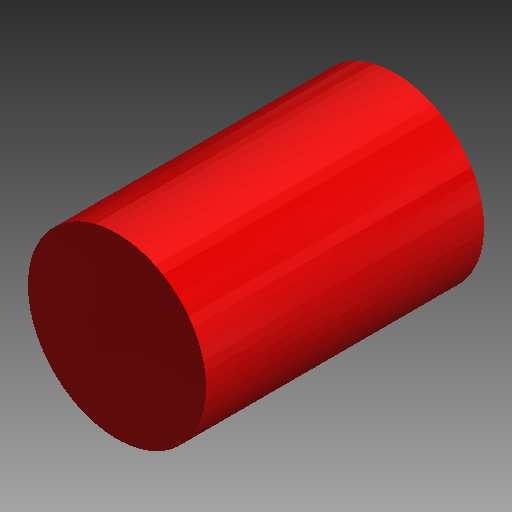
# Autodesk Inventor part: 470uF
Saved by Autodesk Inventor 2018.2 (Build 222227000, 227)
## iProperties
Part Number: 470uF
Material: Generic
Document SubType Name: Modeling
Designer: autocad
Appearance: C12,5-5, 470uF
Author: autocad
Autodesk Inventor part; units mm, degrees
ref_plane "YZ Plane" through (0, 0, 0) normal (1, 0, 0) x (0, 1, 0)
ref_plane "XZ Plane" through (0, 0, 0) normal (0, 1, 0) x (-1, 0, 0)
ref_plane "XY Plane" through (0, 0, 0) normal (0, 0, 1) x (1, 0, 0)
sketch "C12,5-5, 470uF_126" plane through (0, 0, 0) normal (0, 0, 1) x (1, 0, 0)
  line L0 (0.9403, 6.3386) -> (1.557, 6.216)
  line L1 (1.557, 6.216) -> (2.1588, 6.0334)
  line L2 (2.1588, 6.0334) -> (2.7398, 5.7928)
  line L3 (2.7398, 5.7928) -> (3.2944, 5.4963)
  line L4 (3.2944, 5.4963) -> (3.8172, 5.147)
  line L5 (3.8172, 5.147) -> (4.3033, 4.748)
  line L6 (4.3033, 4.748) -> (4.748, 4.3034)
  line L7 (4.748, 4.3034) -> (5.147, 3.8172)
  line L8 (5.147, 3.8172) -> (5.4963, 3.2944)
  line L9 (5.4963, 3.2944) -> (5.7928, 2.7398)
  line L10 (5.7928, 2.7398) -> (6.0334, 2.1588)
  line L11 (6.0334, 2.1588) -> (6.216, 1.557)
  line L12 (6.216, 1.557) -> (6.3386, 0.9403)
  line L13 (6.3386, 0.9403) -> (6.4003, 0.3144)
  line L14 (6.4003, 0.3144) -> (6.4003, 0)
  line L15 (6.4003, 0) -> (6.4003, -0.3144)
  line L16 (6.4003, -0.3144) -> (6.3386, -0.9403)
  line L17 (6.3386, -0.9403) -> (6.216, -1.557)
  line L18 (6.216, -1.557) -> (6.0334, -2.1588)
  line L19 (6.0334, -2.1588) -> (5.7928, -2.7398)
  line L20 (5.7928, -2.7398) -> (5.4963, -3.2944)
  line L21 (5.4963, -3.2944) -> (5.147, -3.8172)
  line L22 (5.147, -3.8172) -> (4.748, -4.3033)
  line L23 (4.748, -4.3033) -> (4.3033, -4.748)
  line L24 (4.3033, -4.748) -> (3.8172, -5.147)
  line L25 (3.8172, -5.147) -> (3.2944, -5.4963)
  line L26 (3.2944, -5.4963) -> (2.7398, -5.7928)
  line L27 (2.7398, -5.7928) -> (2.1588, -6.0334)
  line L28 (2.1588, -6.0334) -> (1.557, -6.216)
  line L29 (1.557, -6.216) -> (0.9403, -6.3386)
  line L30 (0.9403, -6.3386) -> (0.3144, -6.4003)
  line L31 (0.3144, -6.4003) -> (-0.3144, -6.4003)
  line L32 (-0.3144, -6.4003) -> (-0.9403, -6.3386)
  line L33 (-0.9403, -6.3386) -> (-1.557, -6.216)
  line L34 (-1.557, -6.216) -> (-2.1588, -6.0334)
  line L35 (-2.1588, -6.0334) -> (-2.7398, -5.7928)
  line L36 (-2.7398, -5.7928) -> (-3.2944, -5.4963)
  line L37 (-3.2944, -5.4963) -> (-3.8172, -5.147)
  line L38 (-3.8172, -5.147) -> (-4.3034, -4.748)
  line L39 (-4.3034, -4.748) -> (-4.748, -4.3033)
  line L40 (-4.748, -4.3033) -> (-5.147, -3.8172)
  line L41 (-5.147, -3.8172) -> (-5.4963, -3.2944)
  line L42 (-5.4963, -3.2944) -> (-5.7928, -2.7398)
  line L43 (-5.7928, -2.7398) -> (-6.0334, -2.1588)
  line L44 (-6.0334, -2.1588) -> (-6.216, -1.557)
  line L45 (-6.216, -1.557) -> (-6.3386, -0.9403)
  line L46 (-6.3386, -0.9403) -> (-6.4003, -0.3144)
  line L47 (-6.4003, -0.3144) -> (-6.4003, 0)
  line L48 (-6.4003, 0) -> (-6.4003, 0.3144)
  line L49 (-6.4003, 0.3144) -> (-6.3386, 0.9403)
  line L50 (-6.3386, 0.9403) -> (-6.216, 1.557)
  line L51 (-6.216, 1.557) -> (-6.0334, 2.1588)
  line L52 (-6.0334, 2.1588) -> (-5.7928, 2.7398)
  line L53 (-5.7928, 2.7398) -> (-5.4963, 3.2944)
  line L54 (-5.4963, 3.2944) -> (-5.147, 3.8172)
  line L55 (-5.147, 3.8172) -> (-4.748, 4.3034)
  line L56 (-4.748, 4.3034) -> (-4.3034, 4.748)
  line L57 (-4.3034, 4.748) -> (-3.8172, 5.147)
  line L58 (-3.8172, 5.147) -> (-3.2944, 5.4963)
  line L59 (-3.2944, 5.4963) -> (-2.7398, 5.7928)
  line L60 (-2.7398, 5.7928) -> (-2.1588, 6.0334)
  line L61 (-2.1588, 6.0334) -> (-1.557, 6.216)
  line L62 (-1.557, 6.216) -> (-0.9403, 6.3386)
  line L63 (-0.9403, 6.3386) -> (-0.3144, 6.4003)
  line L64 (-0.3144, 6.4003) -> (0.3144, 6.4003)
  line L65 (0.3144, 6.4003) -> (0.9403, 6.3386)
  constraints: 132 end point
extrude "Extrusion1" add sketch "C12,5-5, 470uF_126" along normal blind 20
body "Solid1"
